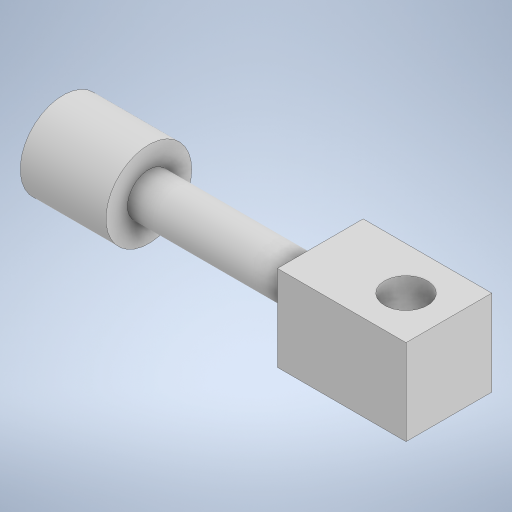
# Autodesk Inventor part: Piston Assembly
Saved by Autodesk Inventor 2023 (Build 270158000, 158)
## iProperties
Created: 2022-12-28
Part Number: Piston Assembly
Material: Generic
Document SubType Name: Modeling
Designer: tgr41
Density: 1 g/cm^3
Appearance: Default
Author: tgr41
Autodesk Inventor part; units mm, degrees
ref_plane "YZ Plane" through (0, 0, 0) normal (1, 0, 0) x (0, 1, 0)
ref_plane "XZ Plane" through (0, 0, 0) normal (0, 1, 0) x (-1, 0, 0)
sketch "Sketch2" plane through (0, 0, 0) normal (0, 1, 0) x (-1, 0, 0)
  line L0 (-25.4, 6.35) -> (-44.45, 6.35)
  line L1 (-44.45, 6.35) -> (-44.45, -6.35)
  line L2 (-44.45, -6.35) -> (-25.4, -6.35)
  line L3 (-25.4, -6.35) -> (-25.4, 6.35)
  line L4 (-25.4, 3.175) -> (-25.4, -3.175) projected
  circle A0 centre (-38.1, 0) radius 3.175
  point P0 (0, 0)
  point P1 (-25.4, 0)
  dimension "d6" = 0
  dimension "d15" = 6.35
  dimension "d16" = 6.35
  dimension "d17" = 12.7
  dimension "d18" = 19.05
  dimension "d19" = 6.35
  constraints: 8 end point, 2 parallel, 1 centre point, 1 horizontal, 1 midpoint, 1 perpendicular
  measures "d6" distance between parallel lines of L3 L4
  measures "d15" diameter of A0
  measures "d16" distance from line of L1 A0.centre
  measures "d17" distance of L0.end L1.end
  measures "d18" distance of L0.start L0.end
  measures "d19" distance from line of L2 A0.centre
extrude "Extrusion1" add sketch "Sketch2" along normal mid plane 12.7
ref_plane "Work Plane2" through (0, 0, 0) normal (0, 1, 0) x (1, 0, 0)
sketch "Sketch4" plane through (0, 0, 0) normal (0, 1, 0) x (1, 0, 0)
  line L0 (25.4, 6.35) -> (25.4, -6.35) projected
  line L1 (25.4, 0) -> (0, 0)
  line L2 (0, 0) -> (0, 3.175)
  line L3 (0, 3.175) -> (25.4, 3.175)
  line L4 (25.4, 0) -> (25.4, 3.175)
  line L5 (0, 0) -> (0, 6.35)
  line L6 (0, 6.35) -> (-12.7, 6.35)
  line L7 (-12.7, 6.35) -> (-12.7, 0)
  line L8 (-12.7, 0) -> (0, 0)
  point P0 (0, 0)
  point P1 (0, 3.175)
  dimension "d20" = 25.4
  dimension "d21" = 3.175
  dimension "d22" = 6.35
  dimension "d23" = 12.7
  constraints: 16 end point, 5 perpendicular, 3 point on line, 1 collinear, 1 horizontal, 1 midpoint
  measures "d20" distance of L1.start L1.end
  measures "d21" distance of L1.end L2.end
  measures "d22" distance of L1.end L5.end
  measures "d23" distance of L5.end L6.end
revolve "Revolution2" add sketch "Sketch4" angle 360 about axis through (25.4, 0, 0) along (-1, 0, 0)
body "Solid1"
